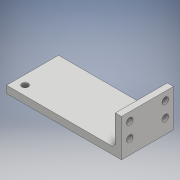
# Autodesk Inventor part: PingCover
Saved by Autodesk Inventor 2018 (Build 220112000, 112)
## iProperties
Created: 2018-08-21
Part Number: PingCover
Material: 一般
Document SubType Name: Modeling
Designer: shun2
Density: 1 g/cm^3
Appearance: 既定
Author: shun2
Autodesk Inventor part; units mm, degrees
ref_plane "YZ Plane" through (0, 0, 0) normal (1, 0, 0) x (0, 1, 0)
ref_plane "XZ Plane" through (0, 0, 0) normal (0, 1, 0) x (-1, 0, 0)
ref_plane "XY Plane" through (0, 0, 0) normal (0, 0, 1) x (1, 0, 0)
sketch "スケッチ2" plane through (0, 0, 0) normal (0, 0, 1) x (1, 0, 0)
  line L0 (22.85, 13.15) -> (-22.85, 13.15)
  line L1 (-22.85, 13.15) -> (-22.85, -8.15)
  line L2 (-22.85, -8.15) -> (22.85, -8.15)
  line L3 (22.85, -8.15) -> (22.85, 13.15)
  circle A0 centre (20.35, 10.65) radius 1.55
  circle A1 centre (-20.35, -5.65) radius 1.55
  circle A2 centre (12.2, 2.5) radius 8.15
  circle A3 centre (-12.2, 2.5) radius 8.15
  line L4 (-2.5, -13.15) -> (-2.5, -8.15)
  line L5 (0, -8.15) -> (0, -13.15)
  line L6 (2.5, -13.15) -> (2.5, -8.15)
  line L7 (-22.85, 15.15) -> (24.9059, 15.15)
  line L8 (-22.85, -10.15) -> (28.1108, -10.15)
  line L9 (-24.85, 8.1193) -> (-24.85, -10.15)
  line L10 (-24.85, 8.1193) -> (-24.85, 15.15)
  line L11 (-24.85, 15.15) -> (28.1108, 15.15)
  line L12 (28.1108, 15.15) -> (28.1108, -10.15)
  line L13 (28.1108, -10.15) -> (-24.85, -10.15)
  line L14 (-24.85, -10.15) -> (-24.85, 15.15)
  point P0 (0, 0)
  point P1 (0, 0)
  constraints: 30 end point, 6 perpendicular, 4 centre point, 3 horizontal, 3 parallel, 2 equal radius, 2 point on line, 1 midpoint, 1 vertical
extrude "押し出し1" add sketch "スケッチ2" along normal blind 3.5 contours L3 L2 L1 L0 | L0 L1 L2 L4 L8 L13 L9 L10 L11 L7 L12 L6 L3 | L6 L8 L5 L2 | L2 L5 L8 L4 | A2 | A3
sketch "スケッチ4" plane through (0, 0, 0) normal (0, 0, -1) x (-1, 0, 0)
  line L0 (-28.1108, -10.15) -> (-28.1108, 15.15) projected
  line L1 (-28.1108, 15.15) -> (-31.1108, 15.15)
  line L2 (-31.1108, 15.15) -> (-31.1108, -10.15)
  line L3 (-31.1108, -10.15) -> (-28.1108, -10.15)
  line L4 (-28.1108, -10.15) -> (-28.1108, 15.15)
  point P0 (0, 0)
  dimension "d3" = 3
  constraints: 8 end point, 2 parallel, 1 horizontal, 1 perpendicular
  measures "d3" distance of L3.end L2.end
extrude "押し出し2" add sketch "スケッチ4" against normal blind 18.3
sketch "スケッチ6" plane through (28.1108, -10.15, 3.5) normal (-1, 0, 0) x (0, 0, 1)
  circle A0 centre (10.8, 21.3) radius 1.6
  circle A1 centre (3.5, 21.3) radius 1.6
  circle A2 centre (10.8, 4) radius 1.6
  circle A3 centre (3.5, 4) radius 1.6
  line L0 (0, 25.3) -> (14.8, 25.3) projected
  line L1 (0, 0) -> (14.8, 0) projected
  line L2 (14.8, 25.3) -> (14.8, 0) projected
  line L3 (0, 25.3) -> (0, 0) projected
  point P0 (-3.5, 10.15)
  dimension "d7" = 3.2
  dimension "d8" = 3.2
  dimension "d9" = 3.2
  dimension "d10" = 3.2
  dimension "d11" = 4
  dimension "d12" = 4
  dimension "d13" = 4
  dimension "d14" = 4
  dimension "d17" = 4
  dimension "d18" = 4
  dimension "d19" = 3.5
  dimension "d20" = 3.5
  constraints: 4 centre point
  measures "d7" diameter of A0
  measures "d8" diameter of A1
  measures "d9" diameter of A2
  measures "d10" diameter of A3
  measures "d11" distance from line of L0 A0.centre
  measures "d12" distance from line of L1 A2.centre
  measures "d13" distance from line of L1 A3.centre
  measures "d14" distance from line of L0 A1.centre
  measures "d17" distance from line of L2 A0.centre
  measures "d18" distance from line of L2 A2.centre
  measures "d19" distance from line of L3 A1.centre
  measures "d20" distance from line of L3 A3.centre
extrude "押し出し3" cut sketch "スケッチ6" against normal blind 3 contours A0 | A1 | A2 | A3
chamfer "面取り1" distance 1.5 angle 45 1 edges at (28.1108, 2.5, 3.5)
